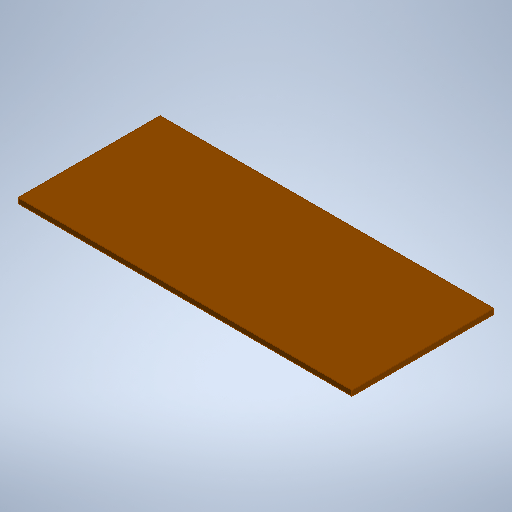
# Autodesk Inventor part: Part1
Saved by Autodesk Inventor 2025.1 (Build 291241000, 241)
## iProperties
Created: 2025-03-06
Part Number: Part1
Material: Plywood, Finish
Document SubType Name: Modeling
Designer: chowg
Density: 0.552 g/cm^3
Appearance: Plywood - New
Category: <PART CATAGORY>
Title: <TITLE>
Author: chowg
Revision Number: 1
Autodesk Inventor part; units mm, degrees
ref_plane "YZ Plane" through (0, 0, 0) normal (1, 0, 0) x (0, 1, 0)
ref_plane "XZ Plane" through (0, 0, 0) normal (0, 1, 0) x (-1, 0, 0)
ref_plane "XY Plane" through (0, 0, 0) normal (0, 0, 1) x (1, 0, 0)
sketch "Sketch6" plane through (0, 0, 0) normal (0, 0, 1) x (1, 0, 0)
  line L0 (0, 0) -> (0, 3)
  line L1 (0, 0) -> (3, 0) construction
  line L2 (0, 3) -> (196.5, 3)
  line L3 (196.5, 3) -> (196.5, 0)
  line L4 (196.5, 0) -> (0, 0)
  dimension "d85" = 3
  dimension "d86" = 90
  dimension "d87" = 196.5
  dimension "d88" = 3
  dimension "d89" = 90
  constraints: 10 end point, 3 perpendicular, 1 horizontal, 1 vertical
  measures "d85" distance of L0.start L0.end
  measures "d86" angle of L1 L0
  measures "d87" distance of L0.end L2.end
  measures "d88" distance of L2.end L3.end
  measures "d89" angle of L2 L3
extrude "Extrusion3" add sketch "Sketch6" along normal blind 83.525
body "Solid2"
